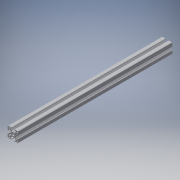
# Autodesk Inventor part: Bosch 30x30
Saved by Autodesk Inventor 2016 (Build 200138000, 138)
## iProperties
Created: 2012-09-30
Part Number: Bosch 30x30
Material: Aluminum 6061
Document SubType Name: Modeling
Designer: Nemo
Density: 1 g/cm^3
Appearance: Aluminum - Flat
Author: Nemo
Autodesk Inventor part; units mm, degrees
ref_plane "YZ Plane" through (0, 0, 0) normal (1, 0, 0) x (0, 1, 0)
ref_plane "XZ Plane" through (0, 0, 0) normal (0, 1, 0) x (-1, 0, 0)
ref_plane "XY Plane" through (0, 0, 0) normal (0, 0, 1) x (1, 0, 0)
sketch "Bosch 30x30 profile" plane through (0, 0, 0) normal (0, 0, 1) x (1, 0, 0)
  arc A0 (-1.4694, 13.3999) -> (-1.1, 15) centre (-4.75, 15) ccw
  arc A1 (-6.3501, 11.7194) -> (-3.1499, 11.7194) centre (-4.75, 15) ccw
  line L0 (-7.8859, 10.4816) -> (-6.3501, 11.7194)
  line L1 (-8.9545, 9) -> (-5.65, 9)
  line L2 (0.7349, 15) -> (1.2545, 15.9)
  line L3 (1.2545, 14.1) -> (0.7349, 15)
  line L4 (-0.2447, 11.8453) -> (-1.4694, 13.3999)
  line L5 (-3.1499, 11.7194) -> (-1.6141, 10.4816)
  line L6 (-5.65, 9) -> (-4.75, 9.5151)
  arc A2 (-1.6141, 10.4816) -> (-0.2447, 11.8453) centre (-4.75, 15) ccw
  line L7 (1.2545, 10.7955) -> (1.2545, 14.1)
  line L8 (-3.85, 9) -> (-0.5455, 9)
  line L9 (-4.75, 9.5151) -> (-3.85, 9)
  line L10 (9.75, 19.25) -> (9.75, 19.35)
  arc A3 (8.05, 19.65) -> (8.65, 19.05) centre (8.65, 19.65) ccw
  line L11 (8.65, 19.05) -> (9.55, 19.05)
  arc A4 (9.55, 19.05) -> (9.75, 19.25) centre (9.55, 19.25) ccw
  arc A5 (8.65, 10.95) -> (8.05, 10.35) centre (8.65, 10.35) ccw
  line L12 (10.05, 10.45) -> (9.95, 10.45)
  line L13 (9.75, 10.65) -> (9.75, 10.75)
  arc A6 (10.25, 10.25) -> (10.05, 10.45) centre (10.05, 10.25) ccw
  arc A7 (9.75, 10.65) -> (9.95, 10.45) centre (9.95, 10.65) ccw
  arc A8 (9.75, 10.75) -> (9.55, 10.95) centre (9.55, 10.75) ccw
  line L14 (9.55, 10.95) -> (8.65, 10.95)
  arc A9 (-1.1, 15) -> (-1.4694, 16.6001) centre (-4.75, 15) ccw
  line L15 (1.2545, 15.9) -> (1.2545, 19.2045)
  line L16 (-1.4694, 16.6001) -> (-0.2447, 18.1547)
  arc A10 (-0.2447, 18.1547) -> (-1.6141, 19.5184) centre (-4.75, 15) ccw
  line L17 (-1.6141, 19.5184) -> (-3.1499, 18.2806)
  arc A11 (-3.1499, 18.2806) -> (-6.3501, 18.2806) centre (-4.75, 15) ccw
  line L18 (-19.55, 19.55) -> (-19.45, 19.55)
  line L19 (-19.25, 19.35) -> (-19.25, 19.25)
  arc A12 (-19.75, 19.75) -> (-19.55, 19.55) centre (-19.55, 19.75) ccw
  arc A13 (-19.25, 19.35) -> (-19.45, 19.55) centre (-19.45, 19.35) ccw
  line L20 (-19.05, 19.05) -> (-18.15, 19.05)
  arc A14 (-19.25, 19.25) -> (-19.05, 19.05) centre (-19.05, 19.25) ccw
  arc A15 (-18.15, 19.05) -> (-17.55, 19.65) centre (-18.15, 19.65) ccw
  arc A16 (-13, 2.4) -> (-12.8, 2.2) centre (-12.8, 2.4) ccw
  line L21 (-13, 4.95) -> (-8.9545, 9)
  line L22 (-9.4, 2.2) -> (-12.8, 2.2)
  line L23 (-9.3, 0.2) -> (-9.3, 0.3)
  arc A17 (-9.5, 0) -> (-9.3, 0.2) centre (-9.5, 0.2) ccw
  arc A18 (-9.1, 0.5) -> (-9.3, 0.3) centre (-9.1, 0.3) ccw
  line L24 (-9.1, 0.5) -> (-9, 0.5)
  line L25 (-8.8, 0.7) -> (-8.8, 1.6)
  arc A19 (-9, 0.5) -> (-8.8, 0.7) centre (-9, 0.7) ccw
  arc A20 (-8.8, 1.6) -> (-9.4, 2.2) centre (-9.4, 1.6) ccw
  arc A21 (-8.0306, 16.6001) -> (-8.0306, 13.3999) centre (-4.75, 15) ccw
  arc A22 (-7.8859, 19.5184) -> (-9.2553, 18.1547) centre (-4.75, 15) ccw
  arc A23 (-9.2553, 11.8453) -> (-7.8859, 10.4816) centre (-4.75, 15) ccw
  line L26 (-9.2553, 18.1547) -> (-8.0306, 16.6001)
  line L27 (-10.7545, 15.9) -> (-10.2349, 15)
  line L28 (-10.2349, 15) -> (-10.7545, 14.1)
  line L29 (-10.7545, 14.1) -> (-10.7545, 10.7955)
  line L30 (-10.7545, 19.2045) -> (-10.7545, 15.9)
  line L31 (-10.7545, 10.7955) -> (-14.8, 6.75)
  line L32 (-14.8, 6.75) -> (-17.35, 6.75)
  arc A24 (-17.55, 6.95) -> (-17.35, 6.75) centre (-17.35, 6.95) ccw
  line L33 (-8.0306, 13.3999) -> (-9.2553, 11.8453)
  line L34 (-0.5455, 21) -> (-3.85, 21)
  line L35 (-3.85, 21) -> (-4.75, 20.4849)
  line L36 (3.5, 25.05) -> (-0.5455, 21)
  line L37 (3.5, 27.6) -> (3.5, 25.05)
  arc A25 (3.5, 27.6) -> (3.3, 27.8) centre (3.3, 27.6) ccw
  line L38 (-4.75, 20.4849) -> (-5.65, 21)
  arc A26 (9.95, 19.55) -> (9.75, 19.35) centre (9.95, 19.35) ccw
  line L39 (9.95, 19.55) -> (10.05, 19.55)
  arc A27 (10.05, 19.55) -> (10.25, 19.75) centre (10.05, 19.75) ccw
  line L40 (8.05, 23.05) -> (8.05, 19.65)
  arc A28 (8.05, 23.05) -> (7.85, 23.25) centre (7.85, 23.05) ccw
  line L41 (1.2545, 19.2045) -> (5.3, 23.25)
  line L42 (5.3, 23.25) -> (7.85, 23.25)
  line L43 (10.25, 19.75) -> (10.25, 28)
  line L44 (-0.4, 29.5) -> (-0.5, 29.5)
  line L45 (-0.2, 29.8) -> (-0.2, 29.7)
  line L46 (-0.7, 29.3) -> (-0.7, 28.4)
  arc A29 (-0.4, 29.5) -> (-0.2, 29.7) centre (-0.4, 29.7) ccw
  arc A30 (0, 30) -> (-0.2, 29.8) centre (0, 29.8) ccw
  arc A31 (-0.5, 29.5) -> (-0.7, 29.3) centre (-0.5, 29.3) ccw
  arc A32 (-0.7, 28.4) -> (-0.1, 27.8) centre (-0.1, 28.4) ccw
  line L47 (8.05, 10.35) -> (8.05, 6.95)
  arc A33 (7.85, 6.75) -> (8.05, 6.95) centre (7.85, 6.95) ccw
  line L48 (7.85, 6.75) -> (5.3, 6.75)
  line L49 (7.95, 5.5) -> (5.75, 5.5)
  line L50 (10.25, 2) -> (10.25, 10.25)
  line L51 (5.3, 6.75) -> (1.2545, 10.7955)
  line L52 (-0.5455, 9) -> (3.5, 4.95)
  arc A34 (5.75, 5.5) -> (4.75, 4.5) centre (5.75, 4.5) ccw
  line L53 (8.95, 2.3) -> (8.95, 4.5)
  line L54 (4.75, 4.5) -> (4.75, 2.3)
  line L55 (3.5, 4.95) -> (3.5, 2.4)
  arc A35 (8.95, 4.5) -> (7.95, 5.5) centre (7.95, 4.5) ccw
  line L56 (-6.3501, 18.2806) -> (-7.8859, 19.5184)
  line L57 (-5.65, 21) -> (-8.9545, 21)
  arc A36 (4.75, 2.3) -> (5.75, 1.3) centre (5.75, 2.3) ccw
  arc A37 (7.95, 1.3) -> (8.95, 2.3) centre (7.95, 2.3) ccw
  line L58 (5.75, 1.3) -> (7.95, 1.3)
  arc A38 (8.25, 0) -> (10.25, 2) centre (8.25, 2) ccw
  arc A39 (3.3, 2.2) -> (3.5, 2.4) centre (3.3, 2.4) ccw
  line L59 (0, 0) -> (8.25, 0)
  line L60 (3.3, 2.2) -> (-0.1, 2.2)
  arc A40 (-0.1, 2.2) -> (-0.7, 1.6) centre (-0.1, 1.6) ccw
  line L61 (-0.5, 0.5) -> (-0.4, 0.5)
  line L62 (-0.2, 0.3) -> (-0.2, 0.2)
  line L63 (-0.7, 1.6) -> (-0.7, 0.7)
  arc A41 (-0.2, 0.3) -> (-0.4, 0.5) centre (-0.4, 0.3) ccw
  arc A42 (-0.2, 0.2) -> (0, 0) centre (0, 0.2) ccw
  arc A43 (-0.7, 0.7) -> (-0.5, 0.5) centre (-0.5, 0.7) ccw
  line L64 (-17.55, 19.65) -> (-17.55, 23.05)
  arc A44 (-17.35, 23.25) -> (-17.55, 23.05) centre (-17.35, 23.05) ccw
  line L65 (-17.35, 23.25) -> (-14.8, 23.25)
  arc A45 (-18.45, 25.5) -> (-17.45, 24.5) centre (-17.45, 25.5) ccw
  line L66 (-17.45, 24.5) -> (-15.25, 24.5)
  line L67 (-19.75, 28) -> (-19.75, 19.75)
  line L68 (-18.45, 27.7) -> (-18.45, 25.5)
  line L69 (-14.8, 23.25) -> (-10.7545, 19.2045)
  arc A46 (-15.25, 24.5) -> (-14.25, 25.5) centre (-15.25, 25.5) ccw
  line L70 (-8.9545, 21) -> (-13, 25.05)
  line L71 (-14.25, 25.5) -> (-14.25, 27.7)
  line L72 (-13, 25.05) -> (-13, 27.6)
  line L73 (5.75, 24.5) -> (7.95, 24.5)
  arc A47 (4.75, 25.5) -> (5.75, 24.5) centre (5.75, 25.5) ccw
  line L74 (-0.1, 27.8) -> (3.3, 27.8)
  line L75 (8.25, 30) -> (0, 30)
  line L76 (8.95, 25.5) -> (8.95, 27.7)
  line L77 (4.75, 27.7) -> (4.75, 25.5)
  arc A48 (5.75, 28.7) -> (4.75, 27.7) centre (5.75, 27.7) ccw
  line L78 (7.95, 28.7) -> (5.75, 28.7)
  arc A49 (8.95, 27.7) -> (7.95, 28.7) centre (7.95, 27.7) ccw
  arc A50 (10.25, 28) -> (8.25, 30) centre (8.25, 28) ccw
  arc A51 (7.95, 24.5) -> (8.95, 25.5) centre (7.95, 25.5) ccw
  arc A52 (-14.25, 27.7) -> (-15.25, 28.7) centre (-15.25, 27.7) ccw
  arc A53 (-17.45, 28.7) -> (-18.45, 27.7) centre (-17.45, 27.7) ccw
  line L79 (-15.25, 28.7) -> (-17.45, 28.7)
  arc A54 (-17.75, 30) -> (-19.75, 28) centre (-17.75, 28) ccw
  arc A55 (-12.8, 27.8) -> (-13, 27.6) centre (-12.8, 27.6) ccw
  line L80 (-9.5, 30) -> (-17.75, 30)
  line L81 (-12.8, 27.8) -> (-9.4, 27.8)
  arc A56 (-9.4, 27.8) -> (-8.8, 28.4) centre (-9.4, 28.4) ccw
  line L82 (-9, 29.5) -> (-9.1, 29.5)
  line L83 (-9.3, 29.7) -> (-9.3, 29.8)
  line L84 (-8.8, 28.4) -> (-8.8, 29.3)
  arc A57 (-8.8, 29.3) -> (-9, 29.5) centre (-9, 29.3) ccw
  arc A58 (-9.3, 29.7) -> (-9.1, 29.5) centre (-9.1, 29.7) ccw
  arc A59 (-9.3, 29.8) -> (-9.5, 30) centre (-9.5, 29.8) ccw
  arc A60 (-18.45, 2.3) -> (-17.45, 1.3) centre (-17.45, 2.3) ccw
  line L85 (-18.45, 4.5) -> (-18.45, 2.3)
  arc A61 (-17.45, 5.5) -> (-18.45, 4.5) centre (-17.45, 4.5) ccw
  arc A62 (-19.75, 2) -> (-17.75, 0) centre (-17.75, 2) ccw
  line L86 (-17.55, 6.95) -> (-17.55, 10.35)
  arc A63 (-17.55, 10.35) -> (-18.15, 10.95) centre (-18.15, 10.35) ccw
  line L87 (-18.15, 10.95) -> (-19.05, 10.95)
  line L88 (-19.25, 10.75) -> (-19.25, 10.65)
  arc A64 (-19.05, 10.95) -> (-19.25, 10.75) centre (-19.05, 10.75) ccw
  arc A65 (-19.45, 10.45) -> (-19.25, 10.65) centre (-19.45, 10.65) ccw
  line L89 (-19.45, 10.45) -> (-19.55, 10.45)
  arc A66 (-19.55, 10.45) -> (-19.75, 10.25) centre (-19.55, 10.25) ccw
  line L90 (-19.75, 10.25) -> (-19.75, 2)
  line L91 (-17.75, 0) -> (-9.5, 0)
  line L92 (-13, 2.4) -> (-13, 4.95)
  arc A67 (-15.25, 1.3) -> (-14.25, 2.3) centre (-15.25, 2.3) ccw
  line L93 (-14.25, 2.3) -> (-14.25, 4.5)
  arc A68 (-14.25, 4.5) -> (-15.25, 5.5) centre (-15.25, 4.5) ccw
  line L94 (-17.45, 1.3) -> (-15.25, 1.3)
  line L95 (-15.25, 5.5) -> (-17.45, 5.5)
  point P0 (-4.7306, 15)
sketch "Sketch1" plane through (0, 0, 0) normal (0, 0, 1) x (1, 0, 0)
  arc A0 (3.2806, -1.6001) -> (3.65, 0) centre (0, 0) ccw
  arc A1 (-1.6001, -3.2806) -> (1.6001, -3.2806) centre (0, 0) ccw
  line L0 (-3.1359, -4.5184) -> (-1.6001, -3.2806)
  line L1 (-4.2045, -6) -> (-0.9, -6)
  line L2 (5.4849, 0) -> (6.0045, 0.9)
  line L3 (6.0045, -0.9) -> (5.4849, 0)
  line L4 (4.5053, -3.1547) -> (3.2806, -1.6001)
  line L5 (1.6001, -3.2806) -> (3.1359, -4.5184)
  line L6 (-0.9, -6) -> (0, -5.4849)
  arc A2 (3.1359, -4.5184) -> (4.5053, -3.1547) centre (0, 0) ccw
  line L7 (6.0045, -4.2045) -> (6.0045, -0.9)
  line L8 (0.9, -6) -> (4.2045, -6)
  line L9 (0, -5.4849) -> (0.9, -6)
  line L10 (14.5, 4.25) -> (14.5, 4.35)
  arc A3 (12.8, 4.65) -> (13.4, 4.05) centre (13.4, 4.65) ccw
  line L11 (13.4, 4.05) -> (14.3, 4.05)
  arc A4 (14.3, 4.05) -> (14.5, 4.25) centre (14.3, 4.25) ccw
  arc A5 (13.4, -4.05) -> (12.8, -4.65) centre (13.4, -4.65) ccw
  line L12 (14.8, -4.55) -> (14.7, -4.55)
  line L13 (14.5, -4.35) -> (14.5, -4.25)
  arc A6 (15, -4.75) -> (14.8, -4.55) centre (14.8, -4.75) ccw
  arc A7 (14.5, -4.35) -> (14.7, -4.55) centre (14.7, -4.35) ccw
  arc A8 (14.5, -4.25) -> (14.3, -4.05) centre (14.3, -4.25) ccw
  line L14 (14.3, -4.05) -> (13.4, -4.05)
  arc A9 (3.65, 0) -> (3.2806, 1.6001) centre (0, 0) ccw
  line L15 (6.0045, 0.9) -> (6.0045, 4.2045)
  line L16 (3.2806, 1.6001) -> (4.5053, 3.1547)
  arc A10 (4.5053, 3.1547) -> (3.1359, 4.5184) centre (0, 0) ccw
  line L17 (3.1359, 4.5184) -> (1.6001, 3.2806)
  arc A11 (1.6001, 3.2806) -> (-1.6001, 3.2806) centre (0, 0) ccw
  line L18 (-14.8, 4.55) -> (-14.7, 4.55)
  line L19 (-14.5, 4.35) -> (-14.5, 4.25)
  arc A12 (-15, 4.75) -> (-14.8, 4.55) centre (-14.8, 4.75) ccw
  arc A13 (-14.5, 4.35) -> (-14.7, 4.55) centre (-14.7, 4.35) ccw
  line L20 (-14.3, 4.05) -> (-13.4, 4.05)
  arc A14 (-14.5, 4.25) -> (-14.3, 4.05) centre (-14.3, 4.25) ccw
  arc A15 (-13.4, 4.05) -> (-12.8, 4.65) centre (-13.4, 4.65) ccw
  arc A16 (-8.25, -12.6) -> (-8.05, -12.8) centre (-8.05, -12.6) ccw
  line L21 (-8.25, -10.05) -> (-4.2045, -6)
  line L22 (-4.65, -12.8) -> (-8.05, -12.8)
  line L23 (-4.55, -14.8) -> (-4.55, -14.7)
  arc A17 (-4.75, -15) -> (-4.55, -14.8) centre (-4.75, -14.8) ccw
  arc A18 (-4.35, -14.5) -> (-4.55, -14.7) centre (-4.35, -14.7) ccw
  line L24 (-4.35, -14.5) -> (-4.25, -14.5)
  line L25 (-4.05, -14.3) -> (-4.05, -13.4)
  arc A19 (-4.25, -14.5) -> (-4.05, -14.3) centre (-4.25, -14.3) ccw
  arc A20 (-4.05, -13.4) -> (-4.65, -12.8) centre (-4.65, -13.4) ccw
  arc A21 (-3.2806, 1.6001) -> (-3.2806, -1.6001) centre (0, 0) ccw
  arc A22 (-3.1359, 4.5184) -> (-4.5053, 3.1547) centre (0, 0) ccw
  arc A23 (-4.5053, -3.1547) -> (-3.1359, -4.5184) centre (0, 0) ccw
  line L26 (-4.5053, 3.1547) -> (-3.2806, 1.6001)
  line L27 (-6.0045, 0.9) -> (-5.4849, 0)
  line L28 (-5.4849, 0) -> (-6.0045, -0.9)
  line L29 (-6.0045, -0.9) -> (-6.0045, -4.2045)
  line L30 (-6.0045, 4.2045) -> (-6.0045, 0.9)
  line L31 (-6.0045, -4.2045) -> (-10.05, -8.25)
  line L32 (-10.05, -8.25) -> (-12.6, -8.25)
  arc A24 (-12.8, -8.05) -> (-12.6, -8.25) centre (-12.6, -8.05) ccw
  line L33 (-3.2806, -1.6001) -> (-4.5053, -3.1547)
  line L34 (4.2045, 6) -> (0.9, 6)
  line L35 (0.9, 6) -> (0, 5.4849)
  line L36 (8.25, 10.05) -> (4.2045, 6)
  line L37 (8.25, 12.6) -> (8.25, 10.05)
  arc A25 (8.25, 12.6) -> (8.05, 12.8) centre (8.05, 12.6) ccw
  line L38 (0, 5.4849) -> (-0.9, 6)
  arc A26 (14.7, 4.55) -> (14.5, 4.35) centre (14.7, 4.35) ccw
  line L39 (14.7, 4.55) -> (14.8, 4.55)
  arc A27 (14.8, 4.55) -> (15, 4.75) centre (14.8, 4.75) ccw
  line L40 (12.8, 8.05) -> (12.8, 4.65)
  arc A28 (12.8, 8.05) -> (12.6, 8.25) centre (12.6, 8.05) ccw
  line L41 (6.0045, 4.2045) -> (10.05, 8.25)
  line L42 (10.05, 8.25) -> (12.6, 8.25)
  line L43 (15, 4.75) -> (15, 13)
  line L44 (4.35, 14.5) -> (4.25, 14.5)
  line L45 (4.55, 14.8) -> (4.55, 14.7)
  line L46 (4.05, 14.3) -> (4.05, 13.4)
  arc A29 (4.35, 14.5) -> (4.55, 14.7) centre (4.35, 14.7) ccw
  arc A30 (4.75, 15) -> (4.55, 14.8) centre (4.75, 14.8) ccw
  arc A31 (4.25, 14.5) -> (4.05, 14.3) centre (4.25, 14.3) ccw
  arc A32 (4.05, 13.4) -> (4.65, 12.8) centre (4.65, 13.4) ccw
  line L47 (12.8, -4.65) -> (12.8, -8.05)
  arc A33 (12.6, -8.25) -> (12.8, -8.05) centre (12.6, -8.05) ccw
  line L48 (12.6, -8.25) -> (10.05, -8.25)
  line L49 (12.7, -9.5) -> (10.5, -9.5)
  line L50 (15, -13) -> (15, -4.75)
  line L51 (10.05, -8.25) -> (6.0045, -4.2045)
  line L52 (4.2045, -6) -> (8.25, -10.05)
  arc A34 (10.5, -9.5) -> (9.5, -10.5) centre (10.5, -10.5) ccw
  line L53 (13.7, -12.7) -> (13.7, -10.5)
  line L54 (9.5, -10.5) -> (9.5, -12.7)
  line L55 (8.25, -10.05) -> (8.25, -12.6)
  arc A35 (13.7, -10.5) -> (12.7, -9.5) centre (12.7, -10.5) ccw
  line L56 (-1.6001, 3.2806) -> (-3.1359, 4.5184)
  line L57 (-0.9, 6) -> (-4.2045, 6)
  arc A36 (9.5, -12.7) -> (10.5, -13.7) centre (10.5, -12.7) ccw
  arc A37 (12.7, -13.7) -> (13.7, -12.7) centre (12.7, -12.7) ccw
  line L58 (10.5, -13.7) -> (12.7, -13.7)
  arc A38 (13, -15) -> (15, -13) centre (13, -13) ccw
  arc A39 (8.05, -12.8) -> (8.25, -12.6) centre (8.05, -12.6) ccw
  line L59 (4.75, -15) -> (13, -15)
  line L60 (8.05, -12.8) -> (4.65, -12.8)
  arc A40 (4.65, -12.8) -> (4.05, -13.4) centre (4.65, -13.4) ccw
  line L61 (4.25, -14.5) -> (4.35, -14.5)
  line L62 (4.55, -14.7) -> (4.55, -14.8)
  line L63 (4.05, -13.4) -> (4.05, -14.3)
  arc A41 (4.55, -14.7) -> (4.35, -14.5) centre (4.35, -14.7) ccw
  arc A42 (4.55, -14.8) -> (4.75, -15) centre (4.75, -14.8) ccw
  arc A43 (4.05, -14.3) -> (4.25, -14.5) centre (4.25, -14.3) ccw
  line L64 (-12.8, 4.65) -> (-12.8, 8.05)
  arc A44 (-12.6, 8.25) -> (-12.8, 8.05) centre (-12.6, 8.05) ccw
  line L65 (-12.6, 8.25) -> (-10.05, 8.25)
  arc A45 (-13.7, 10.5) -> (-12.7, 9.5) centre (-12.7, 10.5) ccw
  line L66 (-12.7, 9.5) -> (-10.5, 9.5)
  line L67 (-15, 13) -> (-15, 4.75)
  line L68 (-13.7, 12.7) -> (-13.7, 10.5)
  line L69 (-10.05, 8.25) -> (-6.0045, 4.2045)
  arc A46 (-10.5, 9.5) -> (-9.5, 10.5) centre (-10.5, 10.5) ccw
  line L70 (-4.2045, 6) -> (-8.25, 10.05)
  line L71 (-9.5, 10.5) -> (-9.5, 12.7)
  line L72 (-8.25, 10.05) -> (-8.25, 12.6)
  line L73 (10.5, 9.5) -> (12.7, 9.5)
  arc A47 (9.5, 10.5) -> (10.5, 9.5) centre (10.5, 10.5) ccw
  line L74 (4.65, 12.8) -> (8.05, 12.8)
  line L75 (13, 15) -> (4.75, 15)
  line L76 (13.7, 10.5) -> (13.7, 12.7)
  line L77 (9.5, 12.7) -> (9.5, 10.5)
  arc A48 (10.5, 13.7) -> (9.5, 12.7) centre (10.5, 12.7) ccw
  line L78 (12.7, 13.7) -> (10.5, 13.7)
  arc A49 (13.7, 12.7) -> (12.7, 13.7) centre (12.7, 12.7) ccw
  arc A50 (15, 13) -> (13, 15) centre (13, 13) ccw
  arc A51 (12.7, 9.5) -> (13.7, 10.5) centre (12.7, 10.5) ccw
  arc A52 (-9.5, 12.7) -> (-10.5, 13.7) centre (-10.5, 12.7) ccw
  arc A53 (-12.7, 13.7) -> (-13.7, 12.7) centre (-12.7, 12.7) ccw
  line L79 (-10.5, 13.7) -> (-12.7, 13.7)
  arc A54 (-13, 15) -> (-15, 13) centre (-13, 13) ccw
  arc A55 (-8.05, 12.8) -> (-8.25, 12.6) centre (-8.05, 12.6) ccw
  line L80 (-4.75, 15) -> (-13, 15)
  line L81 (-8.05, 12.8) -> (-4.65, 12.8)
  arc A56 (-4.65, 12.8) -> (-4.05, 13.4) centre (-4.65, 13.4) ccw
  line L82 (-4.25, 14.5) -> (-4.35, 14.5)
  line L83 (-4.55, 14.7) -> (-4.55, 14.8)
  line L84 (-4.05, 13.4) -> (-4.05, 14.3)
  arc A57 (-4.05, 14.3) -> (-4.25, 14.5) centre (-4.25, 14.3) ccw
  arc A58 (-4.55, 14.7) -> (-4.35, 14.5) centre (-4.35, 14.7) ccw
  arc A59 (-4.55, 14.8) -> (-4.75, 15) centre (-4.75, 14.8) ccw
  arc A60 (-13.7, -12.7) -> (-12.7, -13.7) centre (-12.7, -12.7) ccw
  line L85 (-13.7, -10.5) -> (-13.7, -12.7)
  arc A61 (-12.7, -9.5) -> (-13.7, -10.5) centre (-12.7, -10.5) ccw
  arc A62 (-15, -13) -> (-13, -15) centre (-13, -13) ccw
  line L86 (-12.8, -8.05) -> (-12.8, -4.65)
  arc A63 (-12.8, -4.65) -> (-13.4, -4.05) centre (-13.4, -4.65) ccw
  line L87 (-13.4, -4.05) -> (-14.3, -4.05)
  line L88 (-14.5, -4.25) -> (-14.5, -4.35)
  arc A64 (-14.3, -4.05) -> (-14.5, -4.25) centre (-14.3, -4.25) ccw
  arc A65 (-14.7, -4.55) -> (-14.5, -4.35) centre (-14.7, -4.35) ccw
  line L89 (-14.7, -4.55) -> (-14.8, -4.55)
  arc A66 (-14.8, -4.55) -> (-15, -4.75) centre (-14.8, -4.75) ccw
  line L90 (-15, -4.75) -> (-15, -13)
  line L91 (-13, -15) -> (-4.75, -15)
  line L92 (-8.25, -12.6) -> (-8.25, -10.05)
  arc A67 (-10.5, -13.7) -> (-9.5, -12.7) centre (-10.5, -12.7) ccw
  line L93 (-9.5, -12.7) -> (-9.5, -10.5)
  arc A68 (-9.5, -10.5) -> (-10.5, -9.5) centre (-10.5, -10.5) ccw
  line L94 (-12.7, -13.7) -> (-10.5, -13.7)
  line L95 (-10.5, -9.5) -> (-12.7, -9.5)
  constraints: 1 other
extrude "Extrusion1" add sketch "Sketch1" along normal mid plane 444.5
body "Solid1"
